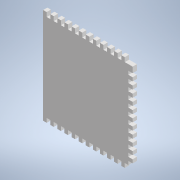
# Autodesk Inventor part: malsten
Saved by Autodesk Inventor 2022 (Build 260153000, 153)
## iProperties
Created: 2023-05-26
Part Number: malsten
Material: Типовые
Document SubType Name: Modeling
Designer: korsh624
Density: 1 g/cm^3
Appearance: По умолчанию
Author: korsh624
Autodesk Inventor part; units mm, degrees
ref_plane "YZ Plane" through (0, 0, 0) normal (1, 0, 0) x (0, 1, 0)
ref_plane "XZ Plane" through (0, 0, 0) normal (0, 1, 0) x (-1, 0, 0)
ref_plane "XY Plane" through (0, 0, 0) normal (0, 0, 1) x (1, 0, 0)
sketch "Эскиз1" plane through (0, 0, 0) normal (0, 0, 1) x (1, 0, 0)
  line L0 (-115, -129) -> (-120, -129) projected
  line L1 (0, -129) -> (-5, -129) projected
  line L2 (-5, -129) -> (-10, -129) projected
  line L3 (-10, -129) -> (-10, -135) projected
  line L4 (-5, -135) -> (-10, -135) projected
  line L5 (-5, -129) -> (-5, -135) projected
  line L6 (-15, -129) -> (-20, -129) projected
  line L7 (-20, -129) -> (-20, -135) projected
  line L8 (-15, -135) -> (-20, -135) projected
  line L9 (-15, -129) -> (-15, -135) projected
  line L10 (-10, -129) -> (-15, -129) projected
  line L11 (-25, -129) -> (-30, -129) projected
  line L12 (-30, -129) -> (-30, -135) projected
  line L13 (-25, -135) -> (-30, -135) projected
  line L14 (-25, -129) -> (-25, -135) projected
  line L15 (-35, -129) -> (-40, -129) projected
  line L16 (-40, -129) -> (-40, -135) projected
  line L17 (-35, -135) -> (-40, -135) projected
  line L18 (-35, -129) -> (-35, -135) projected
  line L19 (-45, -129) -> (-50, -129) projected
  line L20 (-50, -129) -> (-50, -135) projected
  line L21 (-45, -135) -> (-50, -135) projected
  line L22 (-45, -129) -> (-45, -135) projected
  line L23 (-55, -129) -> (-60, -129) projected
  line L24 (-60, -129) -> (-60, -135) projected
  line L25 (-55, -135) -> (-60, -135) projected
  line L26 (-55, -129) -> (-55, -135) projected
  line L27 (-65, -129) -> (-70, -129) projected
  line L28 (-70, -129) -> (-70, -135) projected
  line L29 (-65, -135) -> (-70, -135) projected
  line L30 (-65, -129) -> (-65, -135) projected
  line L31 (-75, -129) -> (-80, -129) projected
  line L32 (-80, -129) -> (-80, -135) projected
  line L33 (-75, -135) -> (-80, -135) projected
  line L34 (-75, -129) -> (-75, -135) projected
  line L35 (-85, -129) -> (-90, -129) projected
  line L36 (-90, -129) -> (-90, -135) projected
  line L37 (-85, -135) -> (-90, -135) projected
  line L38 (-85, -129) -> (-85, -135) projected
  line L39 (-105, -129) -> (-110, -129) projected
  line L40 (-110, -129) -> (-110, -135) projected
  line L41 (-105, -135) -> (-110, -135) projected
  line L42 (-105, -129) -> (-105, -135) projected
  line L43 (-95, -129) -> (-100, -129) projected
  line L44 (-100, -129) -> (-100, -135) projected
  line L45 (-95, -135) -> (-100, -135) projected
  line L46 (-95, -129) -> (-95, -135) projected
  line L47 (-115, -129) -> (-120, -129) projected
  line L48 (-120, -129) -> (-120, -135) projected
  line L49 (-115, -135) -> (-120, -135) projected
  line L50 (-115, -129) -> (-115, -135) projected
  line L51 (-110, -129) -> (-115, -129) projected
  line L52 (-115, 0) -> (-120, 0) projected
  line L53 (-120, 0) -> (-120, -6) projected
  line L54 (-115, -6) -> (-120, -6) projected
  line L55 (-115, 0) -> (-115, -6) projected
  line L56 (-105, 0) -> (-110, 0) projected
  line L57 (-110, 0) -> (-110, -6) projected
  line L58 (-105, -6) -> (-110, -6) projected
  line L59 (-105, 0) -> (-105, -6) projected
  line L60 (-95, 0) -> (-100, 0) projected
  line L61 (-100, 0) -> (-100, -6) projected
  line L62 (-95, -6) -> (-100, -6) projected
  line L63 (-95, 0) -> (-95, -6) projected
  line L64 (-85, 0) -> (-90, 0) projected
  line L65 (-90, 0) -> (-90, -6) projected
  line L66 (-85, -6) -> (-90, -6) projected
  line L67 (-85, 0) -> (-85, -6) projected
  line L68 (-75, 0) -> (-80, 0) projected
  line L69 (-80, 0) -> (-80, -6) projected
  line L70 (-75, -6) -> (-80, -6) projected
  line L71 (-75, 0) -> (-75, -6) projected
  line L72 (-65, 0) -> (-70, 0) projected
  line L73 (-70, 0) -> (-70, -6) projected
  line L74 (-65, -6) -> (-70, -6) projected
  line L75 (-65, 0) -> (-65, -6) projected
  line L76 (-55, 0) -> (-60, 0) projected
  line L77 (-60, 0) -> (-60, -6) projected
  line L78 (-55, -6) -> (-60, -6) projected
  line L79 (-55, 0) -> (-55, -6) projected
  line L80 (-45, 0) -> (-50, 0) projected
  line L81 (-50, 0) -> (-50, -6) projected
  line L82 (-45, -6) -> (-50, -6) projected
  line L83 (-45, 0) -> (-45, -6) projected
  line L84 (-35, -6) -> (-40, -6) projected
  line L85 (-25, 0) -> (-30, 0) projected
  line L86 (-30, 0) -> (-30, -6) projected
  line L87 (-25, -6) -> (-30, -6) projected
  line L88 (-25, 0) -> (-25, -6) projected
  line L89 (-15, 0) -> (-20, 0) projected
  line L90 (-20, 0) -> (-20, -6) projected
  line L91 (-15, -6) -> (-20, -6) projected
  line L92 (-15, 0) -> (-15, -6) projected
  line L93 (-5, 0) -> (-10, 0) projected
  line L94 (-10, 0) -> (-10, -6) projected
  line L95 (-5, -6) -> (-10, -6) projected
  line L96 (-5, 0) -> (-5, -6) projected
  line L97 (0, -6) -> (-5, -6) projected
  line L98 (0, 0) -> (0, -6) projected
  line L99 (0, -6) -> (6, -6) projected
  line L100 (6, 0) -> (6, -6) projected
  line L101 (0, 0) -> (6, 0) projected
  line L102 (0, -6) -> (0, -9) projected
  line L103 (0, -6) -> (0, -9) projected
  line L104 (0, -9) -> (6, -9) projected
  line L105 (6, -6) -> (6, -9) projected
  line L106 (0, -6) -> (6, -6) projected
  line L107 (0, -9) -> (0, -14) projected
  line L108 (0, -14) -> (6, -14) projected
  line L109 (6, -9) -> (6, -14) projected
  line L110 (0, -9) -> (6, -9) projected
  line L111 (0, -19) -> (0, -24) projected
  line L112 (0, -24) -> (6, -24) projected
  line L113 (6, -19) -> (6, -24) projected
  line L114 (0, -19) -> (6, -19) projected
  line L115 (0, -29) -> (0, -34) projected
  line L116 (0, -34) -> (6, -34) projected
  line L117 (6, -29) -> (6, -34) projected
  line L118 (0, -29) -> (6, -29) projected
  line L119 (0, -39) -> (0, -44) projected
  line L120 (0, -44) -> (6, -44) projected
  line L121 (6, -39) -> (6, -44) projected
  line L122 (0, -39) -> (6, -39) projected
  line L123 (0, -49) -> (0, -54) projected
  line L124 (0, -54) -> (6, -54) projected
  line L125 (6, -49) -> (6, -54) projected
  line L126 (0, -49) -> (6, -49) projected
  line L127 (0, -59) -> (0, -64) projected
  line L128 (0, -64) -> (6, -64) projected
  line L129 (6, -59) -> (6, -64) projected
  line L130 (0, -59) -> (6, -59) projected
  line L131 (0, -69) -> (0, -74) projected
  line L132 (0, -74) -> (6, -74) projected
  line L133 (6, -69) -> (6, -74) projected
  line L134 (0, -69) -> (6, -69) projected
  line L135 (0, -79) -> (0, -84) projected
  line L136 (0, -84) -> (6, -84) projected
  line L137 (6, -79) -> (6, -84) projected
  line L138 (0, -79) -> (6, -79) projected
  line L139 (0, -89) -> (0, -94) projected
  line L140 (0, -94) -> (6, -94) projected
  line L141 (6, -89) -> (6, -94) projected
  line L142 (0, -89) -> (6, -89) projected
  line L143 (0, -99) -> (0, -104) projected
  line L144 (0, -104) -> (6, -104) projected
  line L145 (6, -99) -> (6, -104) projected
  line L146 (0, -99) -> (6, -99) projected
  line L147 (0, -109) -> (0, -114) projected
  line L148 (0, -114) -> (6, -114) projected
  line L149 (6, -109) -> (6, -114) projected
  line L150 (0, -109) -> (6, -109) projected
  line L151 (0, -119) -> (0, -124) projected
  line L152 (0, -124) -> (6, -124) projected
  line L153 (6, -119) -> (6, -124) projected
  line L154 (0, -119) -> (6, -119) projected
  line L155 (0, -124) -> (0, -129) projected
  line L156 (-120, -6) -> (0, -6)
  line L157 (0, -6) -> (0, -129)
  line L158 (0, -129) -> (-120, -129)
  line L159 (-120, -129) -> (-120, -6)
  line L160 (-35, 0) -> (-40, 0) projected
  line L161 (-40, 0) -> (-40, -6) projected
  line L162 (-35, -6) -> (-40, -6) projected
  line L163 (-35, 0) -> (-35, -6) projected
  constraints: 4 end point, 1 horizontal, 1 vertical, 6 other
extrude "Выдавливание1" add sketch "Эскиз1" along normal blind 6 contours L50 L49 L48 L0 | L0 L159 L54 L156 L58 L62 L66 L70 L74 L78 L82 L84 L87 L91 L95 L97 L102 L107 L157 L111 L115 L119 L123 L127 L131 L135 L139 L143 L147 L151 L155 L1 L2 L10 L6 L158 L11 L15 L19 L23 L27 L31 L35 L43 L39 L51 | L39 L42 L41 L40 | L53 L52 L55 L54 | L43 L46 L45 L44 | L57 L56 L59 L58 | L35 L38 L37 L36 | L61 L60 L63 L62 | L31 L34 L33 L32 | L65 L64 L67 L66 | L27 L30 L29 L28 | L69 L68 L71 L70 | L23 L26 L25 L24 | L73 L72 L75 L74 | L19 L22 L21 L20 | L77 L76 L79 L78 | L15 L18 L17 L16 | L81 L80 L83 L82 | L11 L14 L13 L12 | L161 L160 L163 L84 | L6 L9 L8 L7 | L86 L85 L88 L87 | L2 L5 L4 L3 | L90 L89 L92 L91 | L94 L93 L96 L95 | L151 L154 L153 L152 | L99 L105 L104 L102 | L147 L150 L149 L148 | L104 L109 L108 L107 | L143 L146 L145 L144 | L114 L113 L112 L111 | L139 L142 L141 L140 | L118 L117 L116 L115 | L135 L138 L137 L136 | L122 L121 L120 L119 | L131 L134 L133 L132 | L126 L125 L124 L123 | L127 L130 L129 L128
sketch "Эскиз2" plane through (0, 0, 6) normal (0, 0, 1) x (1, 0, 0)
  line L0 (0, -6) -> (0, -9) projected
  line L1 (0, -9) -> (6, -9) projected
  line L2 (6, -6) -> (6, -9) projected
  line L3 (0, -6) -> (6, -6) projected
  point P0 (0, 0)
extrude "Выдавливание2" cut sketch "Эскиз2" against normal blind 6
